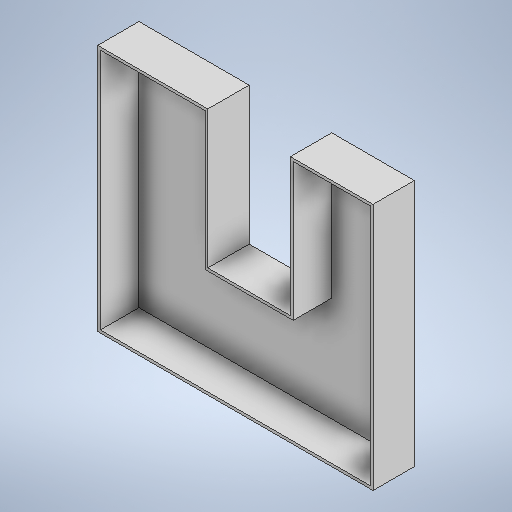
# Autodesk Inventor part: shim
Saved by Autodesk Inventor 2025.2 (Build 292293000, 293)
## iProperties
Created: 2025-02-09
Part Number: shim
Material: Generic
Document SubType Name: Modeling
Designer: kenne
Density: 1 g/cm^3
Appearance: Default
Author: kenne
Autodesk Inventor part; units mm, degrees
ref_plane "YZ Plane" through (0, 0, 0) normal (1, 0, 0) x (0, 1, 0)
ref_plane "XZ Plane" through (0, 0, 0) normal (0, 1, 0) x (-1, 0, 0)
ref_plane "XY Plane" through (0, 0, 0) normal (0, 0, 1) x (1, 0, 0)
sketch "Sketch1" plane through (0, 0, 0) normal (0, 0, 1) x (1, 0, 0)
  line L0 (0, 0) -> (-50, 0) construction
  line L1 (0, 0) -> (50, 0) construction
  line L2 (-50, 0) -> (50, 0)
  line L3 (-50, 0) -> (-50, 90)
  line L4 (-79, 0) -> (-79, 40) construction
  line L5 (-79, 40) -> (-79, 90) construction
  line L6 (-50, 90) -> (-10, 90)
  line L7 (-50, 100.5212) -> (20, 100.5212) construction
  line L8 (-10, 90) -> (-10, 40)
  line L9 (-10, 40) -> (20, 40)
  line L10 (20, 40) -> (20, 90)
  line L11 (20, 90) -> (50, 90)
  line L12 (50, 90) -> (50, 0)
  dimension "d2" = 90
  dimension "d3" = 40
  dimension "d4" = 50
  dimension "d5" = 40
  dimension "d6" = 70
  constraints: 26 end point, 4 horizontal, 4 perpendicular, 3 vertical, 1 collinear, 1 point on line
  measures "d2" distance of L0.end L3.end
  measures "d3" distance of L4.start L4.end
  measures "d4" distance of L4.end L5.end
  measures "d5" distance of L3.end L6.end
  measures "d6" distance of L7.start L7.end
extrude "Extrusion1" add sketch "Sketch1" along normal blind 15
shell "Shell1" thickness 1 removed faces 1 at (-3.3333, 13.3333, 15)
